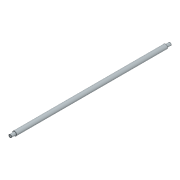
# Autodesk Inventor part: Guías de Vínculo Cabezal
Saved by Autodesk Inventor 2020.3 (Build 243373000, 373)
## iProperties
Created: 2020-05-17
Part Number: Guías de Vínculo Cabezal
Material: Steel, High Strength, Low Alloy
Document SubType Name: Modeling
Designer: Dante
Density: 7.85 g/cm^3
Appearance: Zinc
Mass: 374.214 g
Surface Area: 175.301 cm^2
Volume: 47.6705 cm^3
Author: Dante
Autodesk Inventor part; units mm, degrees
ref_plane "YZ Plane" through (0, 0, 0) normal (1, 0, 0) x (0, 1, 0)
ref_plane "XZ Plane" through (0, 0, 0) normal (0, 1, 0) x (-1, 0, 0)
ref_plane "XY Plane" through (0, 0, 0) normal (0, 0, 1) x (1, 0, 0)
sketch "Sketch1" plane through (0, 0, 0) normal (0, 0, 1) x (1, 0, 0)
  circle A0 centre (0, 0) radius 6
  circle A1 centre (0, 0) radius 3
  dimension "d0" = 12
  dimension "d1" = 6
  constraints: 2 centre point, 2 coincident
  measures "d0" diameter of A0
  measures "d1" diameter of A1
extrude "Extrusion1" add sketch "Sketch1" along normal blind 434 contours A0 | A1
sketch "Sketch2" plane through (0, 0, 434) normal (0, 0, 1) x (1, 0, 0)
  circle A0 centre (0, 0) radius 3
  dimension "d4" = 6
  constraints: 1 centre point, 1 coincident
  measures "d4" diameter of A0
sketch "Sketch3" plane through (0, 0, 0) normal (0, 0, -1) x (-1, 0, 0)
  circle A0 centre (0, 0) radius 3
  dimension "d7" = 6
  constraints: 1 centre point, 1 coincident
  measures "d7" diameter of A0
hole "Agujero1" at (0, 0, 434) direction (0, 0, -1) diameter 6 depth 20 tip angle 118
hole "Agujero2" at (0, 0, 0) direction (0, 0, 1) diameter 6 depth 20 tip angle 118
thread "Rosca3" size "M6x1" class "6H" standard "ISO Metric profile" length 430
thread "Rosca4" size "M6x1" class "6H" standard "ISO Metric profile" length 430
sketch "Sketch4" plane through (0, 0, 434) normal (0, 0, 1) x (1, 0, 0)
  circle A0 centre (0, 0) radius 4
  circle A1 centre (0, 0) radius 6
  dimension "d32" = 8
  constraints: 2 centre point, 2 coincident
  measures "d32" diameter of A0
extrude "Extrusion4" cut sketch "Sketch4" against normal blind 12
sketch "Sketch5" plane through (0, 0, 0) normal (0, 0, -1) x (-1, 0, 0)
  circle A0 centre (0, 0) radius 4
  circle A1 centre (0, 0) radius 6
  dimension "d35" = 8
  constraints: 2 centre point, 1 coincident
  measures "d35" diameter of A0
extrude "Extrusion5" cut sketch "Sketch5" against normal blind 12
body "Solid1"
